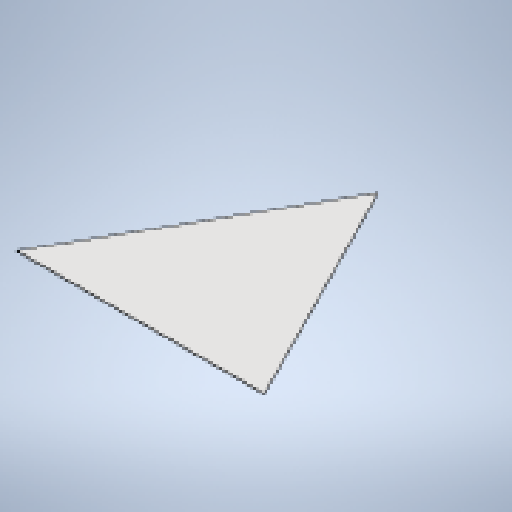
# Autodesk Inventor part: MSC 103 roсket nose
Saved by Autodesk Inventor 2025.1 (Build 291241020, 241B)
## iProperties
Created: 2024-05-19
Part Number: MSC 103 roсket nose
Material: Stainless Steel
Document SubType Name: Sheet Metal
Designer: admin
Density: 8 g/cm^3
Sheet Metal Rule: Default
Sheet Metal Width: 0.000 mm
Sheet Metal Length: 0.000 mm
Sheet Metal Area: 0.000 mm^2
Appearance: Default
Stock Number: МОО 103 ракета нос
Mass: 609.541 g
Surface Area: 1915.65 cm^2
Volume: 76.1926 cm^3
Author: admin
Autodesk Inventor part; units mm, degrees
ref_plane "YZ Plane" through (0, 0, 0) normal (1, 0, 0) x (0, 1, 0)
ref_plane "XZ Plane" through (0, 0, 0) normal (0, 1, 0) x (-1, 0, 0)
ref_plane "XY Plane" through (0, 0, 0) normal (0, 0, 1) x (1, 0, 0)
sketch "Sketch2" plane through (0, 0, 0) normal (0, 0, 1) x (1, 0, 0)
  line L0 (100, 0) -> (-100, 0)
  line L1 (-100, 0) -> (0, 175)
  line L2 (0, 175) -> (100, 0)
  point P0 (0, 0)
  point P1 (0, 0)
  dimension "d8" = 200
  dimension "d9" = 175
  measures "d8" distance of L0.start L0.end
  measures "d9" distance of L1.end point (0, 0)
extrude "Plate1" add sketch "Sketch2" along normal blind 0.8
equation "\"d7\" = Thickness"
equation "\"BendRadius\" = Thickness"
equation "\"BendReliefWidth\" = Thickness"
equation "\"BendReliefDepth\" = 0.5 * Thickness"
equation "\"CornerReliefSize\" = 4 * Thickness"
equation "\"MinimumRemnant\" = 2 * Thickness"
equation "\"TransitionRadius\" = BendRadius"
equation "\"JacobiRadiusSize\" = BendRadius"
equation "\"GapSize\" = Thickness"
equation "\"Thickness\" = 0.8"
body "Solid2"
